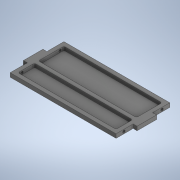
# Autodesk Inventor part: Cockpit_front_frame
Saved by Autodesk Inventor 2020.4 (Build 244396000, 396)
## iProperties
Created: 2022-01-28
Part Number: Cockpit_front_frame
Material: アセタール樹脂、黒
Document SubType Name: Modeling
Designer: Masato Kubotera
Density: 1.425 g/cm^3
Appearance: 滑らか - 黒
Author: Masato Kubotera
Autodesk Inventor part; units mm, degrees
ref_plane "XZ Plane" through (0, 0, 0) normal (0, 1, 0) x (-1, 0, 0)
ref_plane "XY Plane" through (0, 0, 0) normal (0, 0, 1) x (1, 0, 0)
derived "Cockpit_side_frame.ipt"
sketch "スケッチ2" plane through (0, 0, 0) normal (0, 1, 0) x (-1, 0, 0)
  line L0 (-28.5, -22.5) -> (86.5, -22.5) construction
  line L1 (86.5, -22.5) -> (86.5, -138.5)
  line L2 (86.5, -96) -> (-28.5, -96) construction
  line L3 (-28.5, -96) -> (-28.5, -22.5) construction
  line L4 (-28.5, -22.5) -> (86.5, -96) construction
  line L5 (86.5, -22.5) -> (-28.5, -96) construction
  line L6 (36.5, -101) -> (36.5, -133.5)
  line L7 (41.5, -138.5) -> (86.5, -138.5)
  arc A0 (62.6349, -70.4) -> (61.15, -71.8849) centre (61.8925, -71.1425) ccw
  arc A1 (71.15, -72.5349) -> (69.6651, -71.05) centre (70.4075, -71.7925) ccw
  line L8 (63.3349, -71.05) -> (69.6651, -71.05)
  line L9 (62.6349, -70.4) -> (70.3651, -70.4)
  line L10 (61.9, -71.1) -> (71.1, -71.1) construction
  arc A2 (63.3349, -71.05) -> (61.85, -72.5349) centre (62.5925, -71.7925) ccw
  line L11 (61.2, -70.45) -> (71.8, -70.45) construction
  line L12 (71.15, -72.5349) -> (71.15, -83.4651)
  line L13 (71.8, -78) -> (61.2, -78) construction
  line L14 (71.85, -71.8849) -> (71.85, -84.1151)
  line L15 (71.1, -71.1) -> (71.1, -84.9) construction
  line L16 (61.85, -72.5349) -> (61.85, -83.4651)
  line L17 (71.8, -70.45) -> (71.8, -85.55) construction
  line L18 (61.15, -71.8849) -> (61.15, -84.1151)
  line L19 (66.5, -70.45) -> (66.5, -85.55) construction
  line L20 (61.9, -84.9) -> (61.9, -71.1) construction
  line L21 (71.1, -71.1) -> (61.9, -84.9) construction
  line L22 (71.8, -70.45) -> (61.2, -85.55) construction
  line L23 (61.2, -70.45) -> (71.8, -85.55) construction
  line L24 (61.2, -85.55) -> (61.2, -70.45) construction
  line L25 (61.9, -71.1) -> (71.1, -84.9) construction
  arc A3 (71.85, -71.8849) -> (70.3651, -70.4) centre (71.1075, -71.1425) ccw
  line L26 (71.1, -84.9) -> (61.9, -84.9) construction
  line L27 (71.8, -85.55) -> (61.2, -85.55) construction
  arc A4 (61.85, -83.4651) -> (63.3349, -84.95) centre (62.5925, -84.2075) ccw
  arc A5 (61.15, -84.1151) -> (62.6349, -85.6) centre (61.8925, -84.8575) ccw
  line L28 (63.3349, -84.95) -> (69.6651, -84.95)
  line L29 (62.6349, -85.6) -> (70.3651, -85.6)
  arc A6 (69.6651, -84.95) -> (71.15, -83.4651) centre (70.4075, -84.2075) ccw
  arc A7 (70.3651, -85.6) -> (71.85, -84.1151) centre (71.1075, -84.8575) ccw
  line L30 (-23.5, -22.5) -> (-28.5, -27.5)
  line L31 (-28.5, -59.25) -> (86.5, -59.25) construction
  line L32 (29, -22.5) -> (29, -96) construction
  line L33 (-23.5, -96) -> (-28.5, -91)
  line L34 (-28.5, -27.5) -> (-28.5, -91)
  line L35 (-21, -25) -> (-26, -25) construction
  line L36 (-26, -25) -> (-26, -93.5) construction
  line L37 (-26, -93.5) -> (-21, -93.5) construction
  line L38 (-21, -93.5) -> (-21, -25) construction
  line L39 (-21, -25) -> (-26, -93.5) construction
  line L40 (-26, -25) -> (-21, -93.5) construction
  line L41 (-26.05, -46.7) -> (-20.95, -46.7)
  line L42 (-20.95, -46.7) -> (-20.95, -71.8)
  line L43 (-20.95, -71.8) -> (-26.05, -71.8)
  line L44 (-26.05, -71.8) -> (-26.05, -46.7)
  line L45 (-26.05, -46.7) -> (-20.95, -71.8) construction
  line L46 (-20.95, -46.7) -> (-26.05, -71.8) construction
  line L47 (-26, -46.75) -> (-21, -46.75) construction
  line L48 (-26, -71.75) -> (-21, -71.75) construction
  line L49 (-23.5, -25) -> (-23.5, -93.5) construction
  circle A8 centre (-23.5, -35) radius 3
  circle A9 centre (-23.5, -35) radius 1.6
  arc A10 (-24.5651, -46.7) -> (-26.05, -48.1849) centre (-25.3075, -47.4425) ccw
  arc A11 (-20.95, -48.1849) -> (-22.4349, -46.7) centre (-21.6925, -47.4425) ccw
  arc A12 (-22.4349, -71.8) -> (-20.95, -70.3151) centre (-21.6925, -71.0575) ccw
  arc A13 (-26.05, -70.3151) -> (-24.5651, -71.8) centre (-25.3075, -71.0575) ccw
  circle A14 centre (-23.5, -83.5) radius 1.6
  circle A15 centre (-23.5, -83.5) radius 3
  line L50 (31.5, -96) -> (36.5, -101)
  line L51 (-23.5, -96) -> (31.5, -96)
  line L52 (79, -67.5) -> (-21, -67.5) construction
  line L53 (-21, -67.5) -> (-21, -62.5) construction
  line L54 (-21, -62.5) -> (79, -62.5) construction
  line L55 (79, -62.5) -> (79, -67.5) construction
  line L56 (79, -67.5) -> (-21, -62.5) construction
  line L57 (-21, -67.5) -> (79, -62.5) construction
  line L58 (-21, -65) -> (79, -65) construction
  line L59 (29, -62.5) -> (29, -67.5) construction
  line L60 (4, -62.5) -> (4, -67.5) construction
  line L61 (54.05, -62.45) -> (3.95, -62.45)
  line L62 (3.95, -62.45) -> (3.95, -67.55)
  line L63 (3.95, -67.55) -> (54.05, -67.55)
  line L64 (54.05, -67.55) -> (54.05, -62.45)
  line L65 (54.05, -62.45) -> (3.95, -67.55) construction
  line L66 (3.95, -62.45) -> (54.05, -67.55) construction
  arc A16 (5.4349, -62.45) -> (3.95, -63.9349) centre (4.6925, -63.1925) ccw
  circle A17 centre (-3.5, -65) radius 3
  circle A18 centre (-3.5, -65) radius 1.6
  line L67 (54, -62.5) -> (54, -67.5) construction
  arc A19 (54.05, -63.9349) -> (52.5651, -62.45) centre (53.3075, -63.1925) ccw
  circle A20 centre (61.5, -65) radius 3
  circle A21 centre (61.5, -65) radius 1.6
  arc A22 (3.95, -66.0651) -> (5.4349, -67.55) centre (4.6925, -66.8075) ccw
  arc A23 (52.5651, -67.55) -> (54.05, -66.0651) centre (53.3075, -66.8075) ccw
  line L68 (-21, -88.5) -> (79, -88.5) construction
  line L69 (79, -88.5) -> (79, -93.5) construction
  line L70 (79, -93.5) -> (-21, -93.5) construction
  line L71 (-21, -93.5) -> (-21, -88.5) construction
  line L72 (-21, -88.5) -> (79, -93.5) construction
  line L73 (79, -88.5) -> (-21, -93.5) construction
  line L74 (-21, -91) -> (79, -91) construction
  line L75 (29, -88.5) -> (29, -93.5) construction
  line L76 (54.05, -91.05) -> (3.95, -91.05)
  line L77 (3.95, -91.05) -> (3.95, -88.45)
  line L78 (3.95, -88.45) -> (54.05, -88.45)
  line L79 (54.05, -88.45) -> (54.05, -91.05)
  line L80 (54.05, -91.05) -> (3.95, -88.45) construction
  line L81 (3.95, -91.05) -> (54.05, -88.45) construction
  line L82 (4, -88.5) -> (4, -91) construction
  line L83 (54, -88.5) -> (54, -91) construction
  line L84 (4, -89.75) -> (54, -89.75) construction
  arc A24 (6.05, -88.45) -> (3.95, -88.45) centre (5, -88.45) ccw
  arc A25 (54.05, -88.45) -> (51.95, -88.45) centre (53, -88.45) ccw
  arc A26 (51.95, -91.05) -> (54.05, -91.05) centre (53, -91.05) ccw
  arc A27 (3.95, -91.05) -> (6.05, -91.05) centre (5, -91.05) ccw
  circle A28 centre (-3.5, -91) radius 3
  circle A29 centre (-3.5, -91) radius 1.6
  circle A30 centre (61.5, -91) radius 3 construction
  circle A31 centre (61.5, -91) radius 1.6 construction
  line L85 (-23.5, -22.5) -> (64.25, -22.5)
  line L86 (64.25, -22.5) -> (64.25, -17.5)
  line L87 (64.25, -17.5) -> (72.25, -17.5)
  line L88 (72.25, -17.5) -> (72.25, -22.5)
  line L89 (72.25, -22.5) -> (79, -22.5)
  line L90 (79, -22.5) -> (79, -17.5)
  line L91 (86.5, -22.5) -> (86.5, -20)
  line L92 (79, -17.5) -> (84, -17.5)
  line L93 (84, -17.5) -> (86.5, -20)
  line L94 (68.25, -17.5) -> (68.25, -22.5) construction
  arc A32 (62.7651, -22.5) -> (64.25, -21.0151) centre (63.5075, -21.7575) ccw
  arc A33 (72.25, -21.0151) -> (73.7349, -22.5) centre (72.9925, -21.7575) ccw
  arc A34 (77.5151, -22.5) -> (79, -21.0151) centre (78.2575, -21.7575) ccw
  line L95 (-16, -88.5) -> (-16, -68.5) construction
  line L96 (-16, -68.5) -> (64, -68.5) construction
  line L97 (64, -68.5) -> (64, -88.5) construction
  line L98 (45.5, -86) -> (-16.5, -86)
  line L99 (-18.5, -84) -> (-18.5, -72)
  line L100 (-16.5, -70) -> (45.5, -70)
  line L101 (47.5, -72) -> (47.5, -84)
  line L102 (47.5, -86) -> (-18.5, -70) construction
  line L103 (-18.5, -86) -> (47.5, -70) construction
  arc A35 (-16.5, -70) -> (-18.5, -72) centre (-16.5, -72) ccw
  arc A36 (-18.5, -84) -> (-16.5, -86) centre (-16.5, -84) ccw
  arc A37 (45.5, -86) -> (47.5, -84) centre (45.5, -84) ccw
  arc A38 (47.5, -72) -> (45.5, -70) centre (45.5, -72) ccw
  line L104 (36.5, -133.5) -> (41.5, -138.5)
  line L105 (44, -131) -> (39, -131) construction
  line L106 (39, -131) -> (39, -96) construction
  line L107 (39, -96) -> (44, -96) construction
  line L108 (44, -96) -> (44, -131) construction
  line L109 (44, -131) -> (39, -96) construction
  line L110 (39, -131) -> (44, -96) construction
  line L111 (41.5, -96) -> (41.5, -131) construction
  line L112 (39, -113.5) -> (44, -113.5) construction
  line L113 (41.5, -107.5) -> (44, -107.5) construction
  line L114 (41.45, -107.45) -> (44.05, -107.45)
  line L115 (44.05, -107.45) -> (44.05, -119.55)
  line L116 (44.05, -119.55) -> (41.45, -119.55)
  line L117 (41.45, -119.55) -> (41.45, -107.45)
  line L118 (41.45, -107.45) -> (44.05, -119.55) construction
  line L119 (44.05, -107.45) -> (41.45, -119.55) construction
  arc A39 (44.05, -109.55) -> (44.05, -107.45) centre (44.05, -108.5) ccw
  arc A40 (42.9349, -107.45) -> (41.45, -108.9349) centre (42.1925, -108.1925) ccw
  arc A41 (44.05, -119.55) -> (44.05, -117.45) centre (44.05, -118.5) ccw
  line L120 (41.5, -119.5) -> (44, -119.5) construction
  arc A42 (41.45, -118.0651) -> (42.9349, -119.55) centre (42.1925, -118.8075) ccw
  line L121 (42.75, -107.5) -> (42.75, -119.5) construction
  circle A43 centre (41.5, -125.5) radius 3 construction
  circle A44 centre (41.5, -125.5) radius 1.6 construction
  circle A45 centre (41.5, -101.5) radius 3
  circle A46 centre (41.5, -101.5) radius 1.6
  circle A47 centre (-13.5, -55) radius 2
  line L122 (39, -131) -> (77.8645, -131) construction
  line L123 (77.8645, -131) -> (77.8645, -136) construction
  line L124 (77.8645, -136) -> (39, -136) construction
  line L125 (39, -136) -> (39, -131) construction
  line L126 (39, -131) -> (77.8645, -136) construction
  line L127 (77.8645, -131) -> (39, -136) construction
  line L128 (39, -133.5) -> (77.8645, -133.5) construction
  line L129 (58.4322, -131) -> (58.4322, -136) construction
  line L130 (58.4322, -133.5) -> (58.4322, -131) construction
  line L131 (50.8822, -130.95) -> (65.9822, -130.95)
  line L132 (65.9822, -130.95) -> (65.9822, -133.55)
  line L133 (65.9822, -133.55) -> (50.8822, -133.55)
  line L134 (50.8822, -133.55) -> (50.8822, -130.95)
  line L135 (50.8822, -130.95) -> (65.9822, -133.55) construction
  line L136 (65.9822, -130.95) -> (50.8822, -133.55) construction
  line L137 (50.9322, -131) -> (50.9322, -133.5) construction
  arc A48 (52.9822, -130.95) -> (50.8822, -130.95) centre (51.9322, -130.95) ccw
  arc A49 (50.8822, -132.0651) -> (52.3672, -133.55) centre (51.6247, -132.8075) ccw
  arc A50 (65.9822, -130.95) -> (63.8822, -130.95) centre (64.9322, -130.95) ccw
  arc A51 (64.4973, -133.55) -> (65.9822, -132.0651) centre (65.2398, -132.8075) ccw
  line L138 (65.9322, -131) -> (65.9322, -133.5) construction
  line L139 (50.9322, -132.25) -> (65.9322, -132.25) construction
  circle A52 centre (72.4322, -133.5) radius 1.6 construction
  circle A53 centre (72.4322, -133.5) radius 3 construction
  circle A54 centre (44.4322, -133.5) radius 3
  circle A55 centre (44.4322, -133.5) radius 1.6
  line L140 (48.5, -96) -> (77, -96)
  line L141 (79, -98) -> (79, -126.5)
  line L142 (77, -128.5) -> (48.5, -128.5)
  line L143 (46.5, -126.5) -> (46.5, -98)
  line L144 (46.5, -96) -> (79, -128.5) construction
  line L145 (79, -96) -> (46.5, -128.5) construction
  arc A56 (48.5, -96) -> (46.5, -98) centre (48.5, -98) ccw
  arc A57 (46.5, -126.5) -> (48.5, -128.5) centre (48.5, -126.5) ccw
  arc A58 (77, -128.5) -> (79, -126.5) centre (77, -126.5) ccw
  arc A59 (79, -98) -> (77, -96) centre (77, -98) ccw
  line L146 (79, -91.1738) -> (84, -91.1738) construction
  line L147 (84, -91.1738) -> (84, -136) construction
  line L148 (84, -136) -> (79, -136) construction
  line L149 (79, -136) -> (79, -91.1738) construction
  line L150 (79, -91.1738) -> (84, -136) construction
  line L151 (84, -91.1738) -> (79, -136) construction
  line L152 (81.5, -91.1738) -> (81.5, -136) construction
  circle A60 centre (81.5, -93.6738) radius 1.475
  circle A61 centre (81.5, -98.6738) radius 1.475
  circle A62 centre (81.5, -103.6738) radius 1.475
  circle A63 centre (81.5, -133.5) radius 1.6
  arc A64 (84, -91.1738) -> (79, -91.1738) centre (81.5, -133.5) ccw construction
  arc A65 (84.0111, -91.0742) -> (78.9889, -91.0742) centre (81.5, -133.5) ccw construction
  line L153 (86.5, -133.5) -> (81.5, -138.5)
  arc A66 (79, -131) -> (84, -136) centre (81.5, -133.5) ccw construction
  line L154 (79, -65) -> (84, -65) construction
  line L155 (84, -65) -> (84, -91) construction
  line L156 (84, -91) -> (79, -91) construction
  line L157 (79, -91) -> (79, -65) construction
  line L158 (79, -65) -> (84, -91) construction
  line L159 (84, -65) -> (79, -91) construction
  line L160 (79, -78) -> (84, -78) construction
  line L161 (81.5, -65) -> (81.5, -91) construction
  line L162 (79, -73) -> (84, -73) construction
  line L163 (78.95, -72.95) -> (86.5, -72.95)
  line L164 (84.05, -72.95) -> (84.05, -83.05) construction
  line L165 (84.05, -83.05) -> (78.95, -83.05)
  line L166 (78.95, -83.05) -> (78.95, -72.95)
  line L167 (78.95, -72.95) -> (84.05, -83.05) construction
  line L168 (84.05, -72.95) -> (78.95, -83.05) construction
  arc A67 (80.4349, -72.95) -> (78.95, -74.4349) centre (79.6925, -73.6925) ccw
  arc A68 (78.95, -81.5651) -> (80.4349, -83.05) centre (79.6925, -82.3075) ccw
  line L169 (79, -83) -> (84, -83) construction
  circle A69 centre (81.5, -68) radius 1.6
  circle A70 centre (81.5, -68) radius 3
  circle A71 centre (81.5, -88) radius 1.6
  circle A72 centre (81.5, -88) radius 3
  line L170 (84.05, -83.05) -> (86.5, -83.05)
  circle A73 centre (81.5, -133.5) radius 3
  line L171 (75.625, -22.5) -> (75.625, -27.147) construction
  line L172 (60.875, -22.5) -> (60.875, -27.147) construction
  line L173 (64.25, -22.5) -> (72.25, -22.5)
  point P0 (0, 0)
  point P1 (29, -59.25)
  point P2 (-25.7227, -96)
  point P3 (61.85, -71.05)
  point P4 (61.15, -70.4)
  point P5 (66.5, -78)
  point P6 (-23.5, -59.25)
  point P7 (29, -65)
  point P8 (29, -91)
  point P9 (29, -89.75)
  point P10 (29, -89.75)
  point P11 (52.5, -22)
  point P12 (14.5, -78)
  point P13 (-18.5, -61)
  point P14 (47.5, -61)
  point P15 (41.5, -113.5)
  point P16 (42.75, -113.5)
  point P17 (58.4322, -133.5)
  point P18 (58.4322, -132.25)
  point P19 (62.75, -112.25)
  point P20 (81.5, -113.5869)
  point P21 (81.5, -78)
  dimension "d1" = 21
  dimension "d2" = 5
  measures "d1" horizontal distance of L35.start point (0, 0)
  measures "d2" distance of L35.start L35.end
ref_plane "作業平面1" through (21, 0, 0) normal (1, 0, 0) x (0, 1, 0)
sketch "スケッチ3" plane through (21, 0, 0) normal (1, 0, 0) x (0, 1, 0)
  line L0 (-135, -25) -> (0, -25)
  line L1 (0, -25) -> (0, -93.5)
  line L2 (0, -93.5) -> (-135, -93.5)
  line L3 (-135, -93.5) -> (-135, -25)
  line L4 (-135, -25) -> (0, -93.5) construction
  line L5 (0, -25) -> (-135, -93.5) construction
  line L6 (0, -71.75) -> (5, -71.75)
  line L7 (5, -71.75) -> (5, -46.75)
  line L8 (5, -46.75) -> (0, -46.75)
  line L9 (0, -59.25) -> (-135, -59.25) construction
  line L10 (-67.5, -93.5) -> (-67.5, -25)
  arc A0 (1.4849, -71.75) -> (0, -73.2349) centre (0.7425, -72.4925) ccw
  arc A1 (0, -45.2651) -> (1.4849, -46.75) centre (0.7425, -46.0075) ccw
  line L11 (-128, -88.5) -> (-7, -88.5)
  line L12 (-5, -86.5) -> (-5, -69.5)
  line L13 (-7, -67.5) -> (-128, -67.5)
  line L14 (-130, -69.5) -> (-130, -86.5)
  line L15 (-130, -88.5) -> (-5, -67.5) construction
  line L16 (-5, -88.5) -> (-130, -67.5) construction
  line L17 (-128, -30) -> (-7, -30)
  line L18 (-5, -32) -> (-5, -60.5)
  line L19 (-7, -62.5) -> (-128, -62.5)
  line L20 (-130, -60.5) -> (-130, -32)
  line L21 (-130, -30) -> (-5, -62.5) construction
  line L22 (-5, -30) -> (-130, -62.5) construction
  arc A2 (-7, -88.5) -> (-5, -86.5) centre (-7, -86.5) ccw
  arc A3 (-5, -69.5) -> (-7, -67.5) centre (-7, -69.5) ccw
  arc A4 (-128, -67.5) -> (-130, -69.5) centre (-128, -69.5) ccw
  arc A5 (-130, -86.5) -> (-128, -88.5) centre (-128, -86.5) ccw
  arc A6 (-130, -60.5) -> (-128, -62.5) centre (-128, -60.5) ccw
  arc A7 (-7, -62.5) -> (-5, -60.5) centre (-7, -60.5) ccw
  arc A8 (-5, -32) -> (-7, -30) centre (-7, -32) ccw
  arc A9 (-128, -30) -> (-130, -32) centre (-128, -32) ccw
  point P0 (0, 0)
  point P1 (-67.5, -59.25)
  point P2 (0, -67.5)
  point P3 (0, -67.5)
  point P4 (0, -67.5)
  point P5 (0, -62.5)
  point P6 (0, -62.5)
  point P7 (0, -62.5)
  point P8 (-67.5, -78)
  point P9 (-67.5, -46.25)
  point P10 (0, -45.2651)
  point P11 (1.4849, -46.75)
  point P12 (-67.5, -67.5)
  point P13 (-67.5, -88.5)
  point P14 (-67.5, -30)
  point P15 (-67.5, -62.5)
  dimension "d4" = 5
  dimension "d5" = 135
  dimension "d6" = 1.05
  dimension "d7" = 5
  dimension "d8" = 5
  dimension "d9" = 5
  dimension "d10" = 2
  constraints: 44 end point, 21 point on circle, 21 point on line, 16 tangent, 10 centre point, 9 midpoint, 7 equal radius, 6 horizontal, 5 parallel, 3 perpendicular, 3 symmetric about line, 2 coincident, 1 collinear, 1 vertical, 6 other
  measures "d4" distance of L6.start L6.end
  measures "d5" distance of L2.start L2.end
  measures "d6" radius of A0
  measures "d7" horizontal distance of L16.start L2.start
  measures "d8" horizontal distance of L2.start L16.start
  measures "d9" horizontal distance of L0.end L22.start
  measures "d10" radius of A2
extrude "押し出し1" add sketch "スケッチ3" along normal blind 5 contours L0 L1 A1 A0 L2 L10 L11 A2 L12 A3 L13 L19 A7 L18 A8 L17 | L17 A8 L18 A7 L19 L10 | L10 L13 A3 L12 A2 L11 | A1 L8 L7 L6 A0 L1
extrude "押し出し2" cut sketch "スケッチ3" along normal blind 4.5 contours L17 A8 L18 A7 L19 L10 | L10 L13 A3 L12 A2 L11
hole "穴1" at (23.5, 0, -83.5) at (23.5, 0, -35) direction (0, -1, 0) diameter 3.242 depth 5 tip angle 118 thread size "M4x0.7" class "6H" standard "ISO Metric profile"
mirror "ミラー1" about plane through (21, -67.5, -25) normal (0, -1, 0)
equation "\"d7\" = d8"
equation "\"d9\" = d7"
equation "\"d11\" = d2"
equation "\"d3\" = d1"
